Autodesk Inventor part; units mm, degrees
note: some values were not read from the file. Chosen so that the rebuilt part matches the saved one: direction of "Hole2".
(part 10 of 20)
  spline S30 degree 3 poles (-104.40532, -7.588503) (-104.41874, -7.589584) (-104.445196, -7.591715) (-104.484317, -7.593794) (-104.522133, -7.594934) (-104.558443, -7.595019) (-104.593058, -7.594014) (-104.625838, -7.591886) (-104.656702, -7.588699) (-104.685607, -7.584504) (-104.712509, -7.579351) (-104.737369, -7.573293) (-104.760145, -7.566381) (-104.780816, -7.55866) (-104.799541, -7.55008) (-104.816468, -7.540524) (-104.831907, -7.530078) (-104.841054, -7.522069) (-104.845542, -7.518139) knots 0 0 0 0 0.08847523 0.17442408 0.25743028 0.33708941 0.41301484 0.48496567 0.5529194 0.61687848 0.67685349 0.73286663 0.78495643 0.83318442 0.87777974 0.92016243 0.96082909 1 1 1 1
  ellipse E254 centre (-100.14545, -8.274184) end of major axis (-105.576804, -7.705925) minor radius 0.000387 (-103.277546, -7.946168) -> (-105.576804, -7.705925) ccw
  line L389 (-105.263014, -7.451577) -> (-105.576804, -7.705925)
  line L390 (-105.635035, -8.262493) -> (-105.576804, -7.705925)
  spline S31 degree 3 poles (-100.151462, -7.809621) (-100.108876, -7.785381) (-100.024585, -7.737401) (-99.898341, -7.668093) (-99.77384, -7.601642) (-99.611401, -7.517822) (-99.411986, -7.419431) (-99.251066, -7.347613) (-99.172025, -7.312337) knots 0 0 0 0 0.13376268 0.26475964 0.39312605 0.51899363 0.76373828 1 1 1 1
  line L391 (-100.151462, -7.991347) -> (-100.151462, -7.809621)
  line L392 (-93.85162, -7.809621) -> (-93.85162, -7.991347)
  spline S32 degree 3 poles (-94.831057, -7.312337) (-94.752016, -7.347613) (-94.591096, -7.419431) (-94.391681, -7.517822) (-94.229242, -7.601642) (-94.104741, -7.668093) (-93.978497, -7.737401) (-93.894206, -7.785381) (-93.85162, -7.809621) knots 0 0 0 0 0.23626172 0.48100637 0.60687395 0.73524036 0.86623732 1 1 1 1
  line L393 (-99.172025, -7.312337) -> (-94.831057, -7.312337)
  ellipse E255 centre (-97.001541, -7.776601) end of major axis (-101.962541, -7.776601) minor radius 0.5163 (-94.326958, -7.341758) -> (-94.831057, -7.312337) ccw
  ellipse E256 centre (-97.001541, -7.776601) end of major axis (-101.962541, -7.776601) minor radius 0.5163 (-99.172025, -7.312337) -> (-99.676124, -7.341758) ccw
  ellipse E257 centre (-97.001541, -8.273886) end of major axis (-91.540541, -8.273886) minor radius 0.568336 (-91.704205, -8.135789) -> (-93.85162, -7.809621) ccw
  ellipse E258 centre (-97.001541, -8.273886) end of major axis (-102.462541, -8.273886) minor radius 0.568336 (-100.151462, -7.809621) -> (-102.298877, -8.135789) ccw
  line L394 (-90.725538, -7.946169) -> (-90.670456, -8.472633)
  spline S33 degree 3 poles (-91.751687, -7.550801) (-91.669382, -7.577853) (-91.501806, -7.632932) (-91.293188, -7.71057) (-91.122866, -7.777485) (-90.992088, -7.830981) (-90.859278, -7.887152) (-90.770428, -7.926359) (-90.725538, -7.946169) knots 0 0 0 0 0.23621694 0.48094583 0.60681683 0.73519436 0.86621031 1 1 1 1
  spline S34 degree 3 poles (-89.157988, -7.517944) (-89.162657, -7.521949) (-89.172225, -7.530157) (-89.188451, -7.540872) (-89.206369, -7.550757) (-89.226095, -7.559652) (-89.247576, -7.567587) (-89.270807, -7.574535) (-89.295769, -7.580486) (-89.322449, -7.585424) (-89.350849, -7.589337) (-89.381017, -7.592209) (-89.412986, -7.594055) (-89.446759, -7.594893) (-89.48228, -7.594733) (-89.519486, -7.593567) (-89.558321, -7.59147) (-89.584711, -7.589321) (-89.598176, -7.588225) knots 0 0 0 0 0.04039145 0.08278851 0.12750015 0.17478558 0.22486002 0.27790108 0.33405492 0.39344169 0.45616024 0.52241148 0.59256068 0.66658365 0.74441779 0.82598879 0.91121312 1 1 1 1
  ellipse E259 centre (-93.857632, -8.274184) end of major axis (-88.426278, -7.705925) minor radius 0.000387 (-88.426278, -7.705925) -> (-90.725538, -7.946169) ccw
  line L395 (-88.740068, -7.451577) -> (-88.426278, -7.705925)
  line L396 (-88.368047, -8.262493) -> (-88.426278, -7.705925)
  spline S35 degree 3 poles (-102.805515, -6.019471) (-102.76082, -5.999226) (-102.672356, -5.959154) (-102.540099, -5.901692) (-102.409849, -5.846925) (-102.240187, -5.778353) (-102.032335, -5.698687) (-101.865304, -5.641978) (-101.783267, -5.614125) knots 0 0 0 0 0.13378969 0.26480564 0.39318317 0.51905417 0.76378306 1 1 1 1
  line L397 (-102.975863, -7.816663) -> (-102.805515, -6.019471)
  line L398 (-101.783267, -5.614125) -> (-100.987533, -5.689549)
  ellipse E260 centre (-99.622787, -5.818958) end of major axis (-104.561651, -5.350823) minor radius 0.000055 (-104.391855, -5.366902) -> (-104.561651, -5.350823) ccw
  ellipse E261 centre (-99.622787, -5.818958) end of major axis (-104.561651, -5.350823) minor radius 0.000055 (-101.783266, -5.614125) -> (-103.1187, -5.487555) ccw
  spline S36 degree 3 poles (-103.1187, -5.487555) (-103.170269, -5.503399) (-103.271281, -5.534435) (-103.420651, -5.575305) (-103.563643, -5.610313) (-103.699415, -5.638784) (-103.82825, -5.660668) (-103.949867, -5.675145) (-104.046402, -5.680859) (-104.118031, -5.680505) (-104.166268, -5.677754) (-104.210339, -5.672689) (-104.25009, -5.665479) (-104.285402, -5.656276) (-104.324871, -5.642155) (-104.366212, -5.619321) (-104.403393, -5.581425) (-104.424361, -5.534093) (-104.426921, -5.48054) (-104.415741, -5.423604) (-104.400067, -5.386398) (-104.391854, -5.366903) knots 0 0 0 0 0.10413454 0.20397599 0.29888876 0.38827472 0.47171081 0.55106733 0.62459732 0.65820388 0.68929134 0.71781594 0.74378428 0.76721832 0.78816557 0.82463321 0.85738378 0.88888098 0.92222056 0.95924484 1 1 1 1
  ellipse E262 centre (-99.669969, -6.316727) end of major axis (-105.106601, -5.80141) minor radius 0.000061 (-102.805556, -6.019467) -> (-105.106601, -5.80141) ccw
  line L399 (-104.561651, -5.350823) -> (-105.106601, -5.80141)
  ellipse E263 centre (-103.06077, -5.493063) end of major axis (-101.556214, -5.635674) minor radius 0.000017 (-104.392312, -5.366859) -> (-103.201425, -5.479748) ccw
  line L400 (-105.263014, -7.451577) -> (-105.106601, -5.80141)
  spline S37 degree 3 poles (-100.151462, -5.895967) (-100.108876, -5.871702) (-100.024586, -5.823676) (-99.898342, -5.7543) (-99.77384, -5.687785) (-99.611402, -5.603883) (-99.411989, -5.505397) (-99.251066, -5.433507) (-99.172025, -5.398196) knots 0 0 0 0 0.13376751 0.26476787 0.39313627 0.51900446 0.76374629 1 1 1 1
  line L401 (-100.151462, -7.610065) -> (-100.151462, -5.895967)
  line L402 (-93.85162, -5.895967) -> (-93.85162, -7.610065)
  spline S38 degree 3 poles (-94.831057, -5.398196) (-94.752016, -5.433507) (-94.591094, -5.505397) (-94.39168, -5.603883) (-94.229242, -5.687785) (-94.10474, -5.7543) (-93.978496, -5.823676) (-93.894206, -5.871702) (-93.85162, -5.895967) knots 0 0 0 0 0.23625371 0.48099554 0.60686373 0.73523213 0.86623249 1 1 1 1
  line L403 (-99.172025, -5.398196) -> (-94.831057, -5.398196)
  ellipse E264 centre (-97.001541, -5.81898) end of major axis (-101.962541, -5.81898) minor radius 0.467946 (-93.489707, -5.488458) -> (-94.831057, -5.398196) ccw
  ellipse E265 centre (-97.001541, -5.81898) end of major axis (-101.962541, -5.81898) minor radius 0.467946 (-99.172025, -5.398196) -> (-100.513375, -5.488458) ccw
  spline S39 degree 3 poles (-100.513375, -5.488458) (-100.553469, -5.506646) (-100.632452, -5.542475) (-100.749826, -5.59336) (-100.863732, -5.640862) (-100.973727, -5.684603) (-101.079308, -5.724356) (-101.180707, -5.760154) (-101.278249, -5.791822) (-101.371464, -5.819065) (-101.458467, -5.841159) (-101.537132, -5.857069) (-101.605936, -5.86658) (-101.66404, -5.870073) (-101.71224, -5.867867) (-101.750939, -5.859466) (-101.782429, -5.845833) (-101.795976, -5.830244) (-101.802272, -5.822999) knots 0 0 0 0 0.09648314 0.19006443 0.28034292 0.36693478 0.44946267 0.527566 0.60257164 0.67417927 0.74035842 0.79922956 0.84998037 0.89243012 0.92670891 0.95522625 0.97919149 1 1 1 1
  spline S40 degree 3 poles (-92.200822, -5.822993) (-92.206969, -5.830063) (-92.220263, -5.845354) (-92.251449, -5.858818) (-92.290121, -5.867201) (-92.337694, -5.869807) (-92.393667, -5.866938) (-92.458256, -5.858357) (-92.531448, -5.843945) (-92.613159, -5.823884) (-92.702907, -5.798329) (-92.799966, -5.7675) (-92.903601, -5.73162) (-93.013071, -5.690938) (-93.127471, -5.645689) (-93.287624, -5.579321) (-93.408219, -5.525098) (-93.489707, -5.488458) knots 0 0 0 0 0.02031374 0.04393674 0.07255557 0.10706143 0.14790384 0.19530387 0.24973648 0.31134419 0.37967367 0.4542385 0.53453299 0.62003981 0.71019877 0.8041769 1 1 1 1
  ellipse E266 centre (-97.001541, -6.31675) end of major axis (-91.540541, -6.31675) minor radius 0.515109 (-91.846496, -6.146755) -> (-93.85162, -5.895967) ccw
  ellipse E267 centre (-97.001541, -6.31675) end of major axis (-102.462541, -6.31675) minor radius 0.515109 (-100.151462, -5.895967) -> (-102.156586, -6.146755) ccw
  line L404 (-91.197567, -6.019471) -> (-91.027219, -7.816663)
  spline S41 degree 3 poles (-92.219815, -5.614125) (-92.137778, -5.641978) (-91.970747, -5.698687) (-91.762895, -5.778353) (-91.593233, -5.846925) (-91.462983, -5.901692) (-91.330726, -5.959154) (-91.242262, -5.999226) (-91.197567, -6.019471) knots 0 0 0 0 0.23621694 0.48094583 0.60681683 0.73519436 0.86621031 1 1 1 1
  line L405 (-93.015549, -5.689549) -> (-92.219815, -5.614125)
  ellipse E268 centre (-94.380295, -5.818958) end of major axis (-99.319158, -6.287094) minor radius 0.000055 (-90.882926, -5.487417) -> (-92.217961, -5.613949) ccw
  ellipse E269 centre (-94.380295, -5.818958) end of major axis (-89.441431, -5.350823) minor radius 0.000055 (-89.441431, -5.350823) -> (-89.611229, -5.366903) ccw
  spline S42 degree 3 poles (-89.611228, -5.366903) (-89.60278, -5.386911) (-89.58692, -5.424476) (-89.576014, -5.481491) (-89.57887, -5.534018) (-89.599249, -5.58047) (-89.636222, -5.618081) (-89.687727, -5.646719) (-89.753078, -5.66689) (-89.832365, -5.678643) (-89.925655, -5.681717) (-90.032585, -5.676653) (-90.152204, -5.663557) (-90.283105, -5.6426) (-90.423788, -5.613964) (-90.572421, -5.577931) (-90.727128, -5.535824) (-90.83142, -5.503812) (-90.884382, -5.487555) knots 0 0 0 0 0.04184874 0.07857029 0.11114659 0.14190435 0.17426777 0.21118388 0.25459927 0.30565856 0.36551927 0.43456112 0.51220716 0.59775966 0.69045627 0.7893544 0.8930296 1 1 1 1
  ellipse E270 centre (-94.333113, -6.316727) end of major axis (-88.896481, -5.80141) minor radius 0.000061 (-88.896481, -5.80141) -> (-91.197567, -6.019471) ccw
  line L406 (-89.441431, -5.350823) -> (-88.896481, -5.80141)
  line L407 (-88.740068, -7.451577) -> (-88.896481, -5.80141)
  ellipse E271 centre (-99.833277, -5.290471) end of major axis (-103.727023, -4.883084) minor radius 0.000278 (-100.192976, -5.252559) -> (-101.457275, -5.120305) ccw
  ellipse E272 centre (-101.772205, -5.087396) end of major axis (-101.57329, -5.108208) minor radius 0.000014 (-101.663429, -5.098789) -> (-101.57329, -5.108208) ccw
  line L408 (-101.573227, -5.108186) -> (-101.57329, -5.108208)
  ellipse E273 centre (-101.374312, -5.128998) end of major axis (-101.573227, -5.108186) minor radius 0.000014 (-101.457275, -5.120305) -> (-101.573227, -5.108186) ccw
  ellipse E274 centre (-99.833277, -5.290471) end of major axis (-103.180009, -4.940316) minor radius 0.000239 (-101.663429, -5.098789) -> (-103.180009, -4.940316) ccw
  line L409 (-103.180009, -4.940316) -> (-103.236104, -5.476461)
  ellipse E275 centre (-98.189163, 10.423755) end of major axis (-100.436894, 10.658926) minor radius 0.00016 (-100.162743, 10.63032) -> (-100.436894, 10.658926) ccw
  line L410 (-100.436894, 10.658926) -> (-100.733258, 8.711817)
  line L411 (-95.251541, -5.398196) -> (-95.251541, -4.938809)
  ellipse E276 centre (-95.451541, -4.938809) end of major axis (-95.251541, -4.938809) minor radius 0.020814 (-95.251541, -4.938809) -> (-95.368096, -4.919893) ccw
  ellipse E277 centre (-97.001541, -5.290177) end of major axis (-100.916541, -5.290177) minor radius 0.407441 (-95.368096, -4.919893) -> (-98.634987, -4.919893) ccw
  ellipse E278 centre (-95.051541, -4.979583) end of major axis (-95.251541, -4.979583) minor radius 0.020814 (-95.251541, -4.979583) -> (-95.160938, -4.997008) ccw
  ellipse E279 centre (-98.951541, -4.979583) end of major axis (-98.751541, -4.979583) minor radius 0.020814 (-98.842144, -4.997008) -> (-98.751541, -4.979583) ccw
  ellipse E280 centre (-98.551541, -4.938809) end of major axis (-98.751541, -4.938809) minor radius 0.020814 (-98.634987, -4.919893) -> (-98.751541, -4.938809) ccw
  line L412 (-98.751541, -4.938809) -> (-98.751541, -5.398196)
  ellipse E281 centre (-97.001541, -5.290177) end of major axis (-93.636541, -5.290177) minor radius 0.350202 (-93.673685, -5.238287) -> (-95.160938, -4.997008) ccw
  ellipse E282 centre (-97.001541, -5.290177) end of major axis (-100.366541, -5.290177) minor radius 0.350202 (-98.842144, -4.997008) -> (-100.329397, -5.238287) ccw
  ellipse E283 centre (-97.001541, 10.424026) end of major axis (-94.741541, 10.424026) minor radius 0.235202 (-95.963463, 10.632949) -> (-98.039619, 10.632949) ccw
  ellipse E284 centre (-92.62877, -5.128998) end of major axis (-92.429855, -5.108186) minor radius 0.000014 (-92.429855, -5.108186) -> (-92.545807, -5.120305) ccw
  ellipse E285 centre (-94.169805, -5.290471) end of major axis (-98.063552, -5.697857) minor radius 0.000278 (-92.545794, -5.120304) -> (-93.810092, -5.252558) ccw
  line L413 (-92.429792, -5.108208) -> (-92.429855, -5.108186)
  ellipse E286 centre (-92.230877, -5.087396) end of major axis (-92.429792, -5.108208) minor radius 0.000014 (-92.429792, -5.108208) -> (-92.339653, -5.098789) ccw
  ellipse E287 centre (-94.169805, -5.290471) end of major axis (-90.823073, -4.940316) minor radius 0.000239 (-90.823073, -4.940316) -> (-92.339656, -5.098789) ccw
  line L414 (-90.823073, -4.940316) -> (-90.766978, -5.476461)
  ellipse E288 centre (-95.813919, 10.423755) end of major axis (-93.566188, 10.658926) minor radius 0.00016 (-93.566188, 10.658926) -> (-93.840339, 10.63032) ccw
  line L415 (-93.566188, 10.658926) -> (-93.269824, 8.711817)
  ellipse E289 centre (-98.540762, 8.455629) end of major axis (-100.785493, 8.717896) minor radius 0.000114 (-100.027352, 8.629403) -> (-100.785493, 8.717896) ccw
  line L416 (-100.785493, 8.717896) -> (-102.716328, -3.014524)
  line L417 (-102.765192, -3.311436) -> (-103.035733, -4.955341)
  ellipse E290 centre (-97.001541, -7.237173) end of major axis (-100.916541, -7.237173) minor radius 0.45382 (-96.283175, -6.791059) -> (-96.387015, -6.788979) ccw
  ellipse E291 centre (-97.001541, -7.237173) end of major axis (-100.916541, -7.237173) minor radius 0.45382 (-96.660869, -6.785075) -> (-97.397172, -6.785677) ccw
  ellipse E292 centre (-97.001541, -7.237173) end of major axis (-100.916541, -7.237173) minor radius 0.45382 (-97.616067, -6.788979) -> (-97.719907, -6.791059) ccw
  ellipse E293 centre (-97.001541, 8.456315) end of major axis (-94.741541, 8.456315) minor radius 0.261975 (-95.29258, 8.627743) -> (-98.710502, 8.627743) ccw
  ellipse E294 centre (-95.46232, 8.455629) end of major axis (-93.217589, 8.717896) minor radius 0.000114 (-93.217589, 8.717896) -> (-93.97573, 8.629403) ccw
  line L418 (-93.217589, 8.717896) -> (-91.286754, -3.014524)
  line L419 (-91.237891, -3.311436) -> (-90.967349, -4.955341)
  ellipse E295 centre (-97.802609, 13.384052) end of major axis (-97.598523, 13.364708) minor radius 0.000002 (-97.598523, 13.364708) -> (-97.844396, 13.388016) ccw
  ellipse E296 centre (-97.843747, 12.950044) end of major axis (-99.073236, 13.066582) minor radius 0.000014 (-98.187182, 12.98261) -> (-99.073236, 13.066582) ccw
  line L420 (-99.073236, 13.066582) -> (-99.125429, 12.515944)
  arc A2 (-98.1701, 13.394511) -> (-99.073236, 13.066582) centre (-97.983698, 11.473542) ccw
  arc A3 (-97.492698, 13.340033) -> (-97.598523, 13.364708) centre (-97.983698, 11.473542) ccw
  ellipse E297 centre (-99.386879, -3.330114) end of major axis (-103.28441, -2.960682) minor radius 0.000044 (-100.024938, -3.269591) -> (-101.012782, -3.175961) ccw
  ellipse E298 centre (-99.481243, -4.325652) end of major axis (-103.378773, -3.95622) minor radius 0.000044 (-99.731659, -4.301872) -> (-101.107145, -4.171499) ccw
  line L421 (-101.128829, -3.164963) -> (-101.128857, -3.164965)
  line L422 (-101.223192, -4.160501) -> (-101.22322, -4.160503)
  ellipse E299 centre (-99.386879, -3.330114) end of major axis (-102.736864, -3.012582) minor radius 0.000037 (-101.219068, -3.156416) -> (-102.736864, -3.012582) ccw
  ellipse E300 centre (-99.481243, -4.325652) end of major axis (-102.831227, -4.00812) minor radius 0.000037 (-101.31343, -4.151954) -> (-102.589961, -4.030974) ccw
  line L423 (-102.736864, -3.012582) -> (-102.765192, -3.31144)
  ellipse E301 centre (-97.895941, 12.399384) end of major axis (-100.145857, 12.612645) minor radius 0.000025 (-98.980833, 12.502239) -> (-100.145857, 12.612645) ccw
  line L424 (-100.145857, 12.612645) -> (-100.423969, 10.657591)
  ellipse E302 centre (-97.001541, 12.950091) end of major axis (-95.766541, 12.950091) minor radius 0.116491 (-95.815873, 12.982686) -> (-98.187209, 12.982686) ccw
  arc A4 (-97.205699, 13.392747) -> (-97.983204, 13.135272) centre (-97.001541, 11.473583) ccw
  arc A5 (-96.019879, 13.135272) -> (-96.797384, 13.392747) centre (-97.001541, 11.473583) ccw
  ellipse E303 centre (-95.451541, -4.007208) end of major axis (-95.251541, -4.007208) minor radius 0.018865 (-95.251541, -4.007208) -> (-95.368096, -3.990063) ccw
  line L425 (-95.251541, -4.007208) -> (-95.251541, -3.011666)
  ellipse E304 centre (-95.451541, -3.011666) end of major axis (-95.251541, -3.011666) minor radius 0.018865 (-95.251541, -3.011666) -> (-95.368096, -2.994522) ccw
  ellipse E305 centre (-97.001541, -3.330126) end of major axis (-100.916541, -3.330126) minor radius 0.369282 (-95.368096, -2.994522) -> (-98.634987, -2.994522) ccw
  ellipse E306 centre (-97.001541, -4.325668) end of major axis (-100.916541, -4.325668) minor radius 0.369282 (-95.368096, -3.990063) -> (-98.634987, -3.990063) ccw
  ellipse E307 centre (-95.051541, -3.048621) end of major axis (-95.251541, -3.048621) minor radius 0.018865 (-95.251541, -3.048621) -> (-95.160938, -3.064414) ccw
  ellipse E308 centre (-98.951541, -3.048621) end of major axis (-98.751541, -3.048621) minor radius 0.018865 (-98.842144, -3.064414) -> (-98.751541, -3.048621) ccw
  ellipse E309 centre (-98.551541, -3.011666) end of major axis (-98.751541, -3.011666) minor radius 0.018865 (-98.634987, -2.994522) -> (-98.751541, -3.011666) ccw
  ellipse E310 centre (-98.551541, -4.007208) end of major axis (-98.751541, -4.007208) minor radius 0.018865 (-98.634987, -3.990063) -> (-98.751541, -4.007208) ccw
  line L426 (-98.751541, -3.011666) -> (-98.751541, -4.007208)
  ellipse E311 centre (-95.051541, -4.044163) end of major axis (-95.251541, -4.044163) minor radius 0.018865 (-95.251541, -4.044163) -> (-95.160938, -4.059955) ccw
  line L427 (-95.251541, -4.044163) -> (-95.251541, -4.007208)
  ellipse E312 centre (-98.951541, -4.044163) end of major axis (-98.751541, -4.044163) minor radius 0.018865 (-98.842144, -4.059955) -> (-98.751541, -4.044163) ccw
  line L428 (-98.751541, -4.007208) -> (-98.751541, -4.044163)
  ellipse E313 centre (-97.001541, -3.330126) end of major axis (-93.636541, -3.330126) minor radius 0.317404 (-93.750966, -3.248059) -> (-95.160938, -3.064414) ccw
  ellipse E314 centre (-97.001541, -3.330126) end of major axis (-100.366541, -3.330126) minor radius 0.317404 (-98.842144, -3.064414) -> (-100.252116, -3.248059) ccw
  ellipse E315 centre (-97.001541, -4.325668) end of major axis (-100.366541, -4.325668) minor radius 0.317404 (-100.271387, -4.25072) -> (-100.340805, -4.286487) ccw
  ellipse E316 centre (-97.001541, -4.325668) end of major axis (-93.636541, -4.325668) minor radius 0.317404 (-98.842144, -4.059955) -> (-100.062388, -4.1938) ccw
  ellipse E317 centre (-97.001541, -4.325668) end of major axis (-93.636541, -4.325668) minor radius 0.317404 (-93.940694, -4.1938) -> (-95.160938, -4.059955) ccw
  ellipse E318 centre (-97.001541, -4.325668) end of major axis (-93.636541, -4.325668) minor radius 0.317404 (-93.662277, -4.286487) -> (-93.731695, -4.25072) ccw
  ellipse E319 centre (-97.001541, 12.399429) end of major axis (-94.741541, 12.399429) minor radius 0.213175 (-95.021924, 12.50227) -> (-98.981158, 12.50227) ccw
  ellipse E320 centre (-96.200474, 13.384052) end of major axis (-96.404559, 13.364708) minor radius 0.000002 (-96.158686, 13.388016) -> (-96.404559, 13.364708) ccw
  ellipse E321 centre (-96.159336, 12.950044) end of major axis (-94.929846, 13.066582) minor radius 0.000014 (-94.929846, 13.066582) -> (-95.8159, 12.98261) ccw
  line L429 (-94.929846, 13.066582) -> (-94.877653, 12.515944)
  arc A6 (-96.404559, 13.364708) -> (-96.510384, 13.340033) centre (-96.019384, 11.473542) ccw
  arc A7 (-94.929846, 13.066582) -> (-95.832982, 13.394511) centre (-96.019384, 11.473542) ccw
  ellipse E322 centre (-94.616203, -3.330114) end of major axis (-98.513733, -3.699546) minor radius 0.000044 (-92.989786, -3.175912) -> (-93.977586, -3.269538) ccw
  ellipse E323 centre (-94.521839, -4.325652) end of major axis (-98.41937, -4.695083) minor radius 0.000044 (-92.895423, -4.17145) -> (-94.270859, -4.301818) ccw
  line L430 (-92.874225, -3.164965) -> (-92.874253, -3.164963)
  line L431 (-92.779862, -4.160503) -> (-92.77989, -4.160501)
  ellipse E324 centre (-94.616203, -3.330114) end of major axis (-91.266218, -3.012582) minor radius 0.000037 (-91.266218, -3.012582) -> (-92.784108, -3.156425) ccw
  ellipse E325 centre (-94.521839, -4.325652) end of major axis (-91.171855, -4.00812) minor radius 0.000037 (-91.41312, -4.030974) -> (-92.68965, -4.151954) ccw
  line L432 (-91.266218, -3.012582) -> (-91.23789, -3.31144)
  ellipse E326 centre (-96.107141, 12.399384) end of major axis (-93.857225, 12.612645) minor radius 0.000025 (-93.857225, 12.612645) -> (-95.022249, 12.502239) ccw
  line L433 (-93.857225, 12.612645) -> (-93.579113, 10.657591)
  line L434 (-89.836306, -39.801561) -> (-90.501958, -38.086358)
  line L435 (-87.761586, -39.801561) -> (-88.303845, -37.920957)
  line L436 (-106.795587, -39.801561) -> (-106.897672, -37.782333)
  line L437 (-104.725301, -39.801561) -> (-104.622766, -37.850618)
  line L438 (-89.880813, -39.139047) -> (-90.11399, -38.038909)
  line L439 (-87.749763, -39.085429) -> (-87.891287, -37.830541)
  line L440 (-106.253319, -39.085429) -> (-106.111795, -37.830541)
  line L441 (-104.12227, -39.139047) -> (-103.889092, -38.038909)
  line L442 (-89.277781, -39.801561) -> (-89.380316, -37.850618)
  line L443 (-87.207496, -39.801561) -> (-87.106374, -37.801401)
  line L444 (-106.241496, -39.801561) -> (-105.696994, -37.913178)
  line L445 (-104.166776, -39.801561) -> (-103.501124, -38.086358)
  line L446 (-89.601791, -38.390849) -> (-89.684484, -37.945244)
  line L447 (-87.415885, -38.40542) -> (-87.476578, -37.784138)
  line L448 (-106.587197, -38.40542) -> (-106.526504, -37.784138)
  line L449 (-104.401292, -38.390849) -> (-104.318598, -37.945244)
  ellipse E327 centre (-107.424482, -24.551038) end of major axis (-107.497848, -24.375774) minor radius 0.172083 (-107.599289, -24.542874) -> (-107.493364, -24.717688) ccw
  ellipse E328 centre (-107.483138, -24.575592) end of major axis (-107.409772, -24.750856) minor radius 0.172083 (-107.618457, -24.683795) -> (-107.56024, -24.737582) ccw
  ellipse E329 centre (-107.413108, -27.354914) end of major axis (-107.486474, -27.17965) minor radius 0.172083 (-107.525342, -27.203052) -> (-107.545513, -27.222774) ccw
  ellipse E330 centre (-107.674507, -24.573932) end of major axis (-107.683372, -24.763725) minor radius 0.073999 (-107.669789, -24.761191) -> (-107.600209, -24.542831) ccw
  ellipse E331 centre (-107.812513, -24.567486) end of major axis (-107.821377, -24.757279) minor radius 0.073999 (-107.807794, -24.754746) -> (-107.738215, -24.536385) ccw
  ellipse E332 centre (-107.742483, -27.346808) end of major axis (-107.733618, -27.157015) minor radius 0.073999 (-107.668184, -27.315707) -> (-107.747201, -27.159549) ccw
  ellipse E333 centre (-107.354452, -27.33036) end of major axis (-107.427818, -27.155096) minor radius 0.172083 (-107.458618, -27.172309) -> (-107.529259, -27.322196) ccw
  ellipse E334 centre (-107.604477, -27.353254) end of major axis (-107.595612, -27.163461) minor radius 0.073999 (-107.530179, -27.322153) -> (-107.595612, -27.163461) ccw
  line L450 (-107.595612, -27.163461) -> (-107.733618, -27.157015)
  line L451 (-107.320508, -24.770227) -> (-107.411556, -24.765974)
  line L452 (-107.337736, -24.742129) -> (-107.218796, -24.747684)
  line L453 (-106.733437, -27.012581) -> (-106.744387, -26.578006)
  line L454 (-106.779637, -25.17899) -> (-106.784594, -24.982296)
  line L455 (-108.045478, -24.854241) -> (-107.807794, -24.754746)
  line L456 (-107.669789, -24.761191) -> (-107.800448, -24.815885)
  line L457 (-107.747201, -27.159549) -> (-107.847783, -27.201653)
  line L458 (-108.068664, -27.10488) -> (-108.119821, -25.074595)
  line L459 (-107.151556, -27.152798) -> (-107.232991, -27.148994)
  line L460 (-107.981815, -25.081041) -> (-107.930658, -27.111326)
  line L461 (-106.725937, -24.957742) -> (-106.720023, -25.192452)
  line L462 (-106.694116, -26.22064) -> (-106.67478, -26.988027)
  ellipse E335 centre (-107.517905, -23.195787) end of major axis (-107.591271, -23.020523) minor radius 0.172083 (-107.591271, -23.020523) -> (-107.650311, -23.063647) ccw
  ellipse E336 centre (-107.378341, -28.734719) end of major axis (-107.304975, -28.909983) minor radius 0.172083 (-107.51366, -28.842922) -> (-107.50192, -28.857667) ccw
  ellipse E337 centre (-107.319685, -28.710166) end of major axis (-107.393051, -28.534902) minor radius 0.172083 (-107.494492, -28.702001) -> (-107.434983, -28.842027) ccw
  ellipse E338 centre (-107.459249, -23.171233) end of major axis (-107.532615, -22.995969) minor radius 0.172083 (-107.51781, -22.990633) -> (-107.634056, -23.163068) ccw
  line L463 (-107.591271, -23.020523) -> (-107.532615, -22.995969)
  line L464 (-107.351927, -28.922992) -> (-106.338665, -28.970317)
  line L465 (-107.494492, -28.702001) -> (-107.529259, -27.322196)
  line L466 (-106.927292, -28.915532) -> (-107.278106, -28.899146)
  line L467 (-107.250149, -22.99396) -> (-107.201576, -22.996229)
  line L468 (-107.599289, -24.542874) -> (-107.634056, -23.163068)
  ellipse E339 centre (-106.908244, -27.004416) end of major axis (-106.834878, -27.17968) minor radius 0.172083 (-106.768249, -27.127038) -> (-106.733437, -27.012581) ccw
  ellipse E340 centre (-106.959401, -24.974131) end of major axis (-106.886035, -25.149395) minor radius 0.172083 (-106.784594, -24.982296) -> (-106.792606, -24.930572) ccw
  ellipse E341 centre (-107.994366, -27.073779) end of major axis (-108.00323, -27.263572) minor radius 0.073999 (-108.068664, -27.10488) -> (-108.052515, -27.206678) ccw
  ellipse E342 centre (-108.045523, -25.043494) end of major axis (-108.036658, -24.853701) minor radius 0.073999 (-108.063135, -24.864536) -> (-108.119821, -25.074595) ccw
  ellipse E343 centre (-106.900744, -24.949578) end of major axis (-106.97411, -24.774314) minor radius 0.172083 (-106.725937, -24.957742) -> (-106.753988, -24.858996) ccw
  ellipse E344 centre (-106.849587, -26.979863) end of major axis (-106.776221, -27.155126) minor radius 0.172083 (-106.734412, -27.129255) -> (-106.67478, -26.988027) ccw
  ellipse E345 centre (-107.85636, -27.080224) end of major axis (-107.847495, -26.890431) minor radius 0.073999 (-107.930658, -27.111326) -> (-107.920556, -27.192393) ccw
  ellipse E346 centre (-107.907517, -25.049939) end of major axis (-107.898652, -24.860146) minor radius 0.073999 (-107.97813, -25.008291) -> (-107.981815, -25.081041) ccw
  line L469 (-107.738215, -24.536385) -> (-107.772982, -23.15658)
  line L470 (-107.851998, -23.000422) -> (-108.036921, -23.077831)
  line L471 (-108.14986, -29.100931) -> (-107.702997, -28.913873)
  line L472 (-107.633418, -28.695512) -> (-107.668184, -27.315707)
  line L473 (-107.600209, -24.542831) -> (-107.634976, -23.163025)
  line L474 (-107.495412, -28.701958) -> (-107.530179, -27.322153)
  line L475 (-108.417464, -29.277166) -> (-107.564992, -28.920319)
  ellipse E347 centre (-107.84728, -23.187681) end of major axis (-107.838415, -22.997888) minor radius 0.073999 (-107.772982, -23.15658) -> (-107.851998, -23.000422) ccw
  ellipse E348 centre (-107.707716, -28.726614) end of major axis (-107.71658, -28.916407) minor radius 0.073999 (-107.702997, -28.913873) -> (-107.633418, -28.695512) ccw
  ellipse E349 centre (-107.709274, -23.194127) end of major axis (-107.70041, -23.004334) minor radius 0.073999 (-107.634976, -23.163025) -> (-107.70041, -23.004334) ccw
  ellipse E350 centre (-107.56971, -28.733059) end of major axis (-107.578575, -28.922853) minor radius 0.073999 (-107.564992, -28.920319) -> (-107.495412, -28.701958) ccw
  line L476 (-107.838415, -22.997888) -> (-107.70041, -23.004334)
  line L477 (-107.648967, -29.358549) -> (-108.285216, -29.328832)
  line L478 (-108.343872, -29.353386) -> (-107.647584, -29.385907)
  ellipse E351 centre (-108.187455, -29.287909) end of major axis (-108.437376, -29.294207) minor radius 0.041852 (-108.417464, -29.277166) -> (-108.285216, -29.328832) ccw
  ellipse E352 centre (-108.187455, -29.287909) end of major axis (-108.587328, -29.297985) minor radius 0.066962 (-108.585467, -29.291196) -> (-108.343872, -29.353386) ccw
  line L479 (-108.587477, -29.292074) -> (-108.587328, -29.297985)
  line L480 (-87.560521, -24.714054) -> (-87.279601, -24.703624)
  line L481 (-87.428378, -26.95356) -> (-87.56132, -25.684022)
  ellipse E353 centre (-87.393205, -23.121791) end of major axis (-87.418109, -22.93343) minor radius 0.101721 (-87.313826, -23.0264) -> (-87.412975, -22.932997) ccw
  line L482 (-87.412975, -22.932997) -> (-87.516236, -22.93683)
  line L483 (-87.324785, -28.914822) -> (-87.030053, -28.903879)
  line L484 (-87.019614, -28.903492) -> (-86.951072, -28.900947)
  line L485 (-87.511613, -28.933701) -> (-87.405313, -28.929755)
  ellipse E354 centre (-87.326403, -26.949774) end of major axis (-87.301499, -27.138135) minor radius 0.101721 (-87.428378, -26.95356) -> (-87.338805, -27.130661) ccw
  ellipse E355 centre (-87.540751, -24.902848) end of major axis (-87.565655, -24.714488) minor radius 0.101721 (-87.560521, -24.714054) -> (-87.560874, -24.714068) ccw
  line L486 (-106.375782, -22.953277) -> (-106.465761, -22.953134)
  line L487 (-106.710484, -28.915657) -> (-106.670867, -28.91572)
  line L488 (-106.481887, -28.916019) -> (-106.25106, -28.916385)
  line L489 (-106.158165, -28.727707) -> (-106.085563, -28.034397)
  line L490 (-106.587235, -28.932506) -> (-106.518088, -28.932616)
  ellipse E356 centre (-106.23129, -28.727591) end of major axis (-106.254421, -28.916178) minor radius 0.072673 (-106.25106, -28.916385) -> (-106.158165, -28.727707) ccw
  line L491 (-106.219982, -27.147438) -> (-106.263661, -27.147368)
  ellipse E357 centre (-106.098926, -22.998128) end of major axis (-106.496751, -22.956469) minor radius 0.017093 (-106.465761, -22.953134) -> (-106.496751, -22.956469) ccw
  line L492 (-106.496751, -22.956469) -> (-106.497264, -22.961369)
  line L493 (-85.58781, -29.276018) -> (-85.977019, -29.308696)
  line L494 (-86.35471, -29.370329) -> (-85.506315, -29.299099)
  ellipse E358 centre (-85.583091, -29.088759) end of major axis (-85.634867, -29.271568) minor radius 0.156811 (-85.58781, -29.276018) -> (-85.503367, -29.241082) ccw
  ellipse E359 centre (-85.501597, -29.11184) end of major axis (-85.553373, -29.294649) minor radius 0.156811 (-85.506315, -29.299099) -> (-85.419544, -29.262283) ccw
  line L495 (-86.327432, -23.005815) -> (-86.358769, -22.996939)
  line L496 (-86.50777, -28.910391) -> (-86.068015, -29.03494)
  line L497 (-86.515336, -28.954467) -> (-85.449259, -29.256406)
  line L498 (-86.402973, -24.751263) -> (-86.087861, -24.840511)
  line L499 (-85.989353, -25.057006) -> (-86.04051, -27.087291)
  ellipse E360 centre (-86.738642, -24.779445) end of major axis (-86.338769, -24.789521) minor radius 0.066962 (-86.402973, -24.751263) -> (-86.627877, -24.717796) ccw
  line L500 (-87.36115, -24.751914) -> (-87.020704, -24.723331)
  ellipse E361 centre (-86.738642, -24.779445) end of major axis (-86.988563, -24.773148) minor radius 0.041852 (-86.754457, -24.737277) -> (-86.868524, -24.740497) ccw
  line L501 (-86.372358, -24.806153) -> (-86.437773, -24.787626)
  ellipse E362 centre (-86.799236, -27.184249) end of major axis (-87.199109, -27.174173) minor radius 0.066962 (-86.473415, -27.153396) -> (-86.748949, -27.119029) ccw
  line L502 (-87.458214, -24.97685) -> (-87.464599, -25.230258)
  ellipse E363 centre (-86.092579, -25.02777) end of major axis (-86.108475, -24.838436) minor radius 0.102463 (-85.989353, -25.057006) -> (-86.087861, -24.840511) ccw
  ellipse E364 centre (-86.143736, -27.058055) end of major axis (-86.159632, -26.868721) minor radius 0.102463 (-86.068434, -27.202124) -> (-86.04051, -27.087291) ccw
  ellipse E365 centre (-87.298771, -24.963464) end of major axis (-87.246995, -24.780654) minor radius 0.156811 (-87.447033, -24.912144) -> (-87.458214, -24.97685) ccw
  ellipse E366 centre (-87.380266, -24.940382) end of major axis (-87.432042, -25.123192) minor radius 0.156811 (-87.415314, -24.762322) -> (-87.5126, -24.851792) ccw
  line L503 (-87.666452, -28.957799) -> (-87.369579, -28.932874)
  line L504 (-87.037597, -28.905002) -> (-86.979263, -28.900104)
  ellipse E367 centre (-86.843439, -28.938573) end of major axis (-86.593519, -28.94487) minor radius 0.041852 (-86.834301, -28.89696) -> (-86.979263, -28.900104) ccw
  ellipse E368 centre (-86.694439, -23.025121) end of major axis (-87.094312, -23.015046) minor radius 0.066962 (-86.358769, -22.996939) -> (-86.662307, -22.959142) ccw
  ellipse E369 centre (-86.843439, -28.938573) end of major axis (-87.243312, -28.928497) minor radius 0.066962 (-86.50777, -28.910391) -> (-86.672405, -28.882215) ccw
  ellipse E370 centre (-85.444541, -29.069147) end of major axis (-85.428645, -29.258481) minor radius 0.102463 (-85.449259, -29.256406) -> (-85.430097, -29.258583) ccw
  line L505 (-87.934435, -29.313625) -> (-87.978745, -29.301075)
  ellipse E371 centre (-107.762483, -24.584082) end of major axis (-107.838534, -24.409967) minor radius 0.168992 (-107.934755, -24.578254) -> (-107.844467, -24.740213) ccw
  ellipse E372 centre (-107.825313, -24.611525) end of major axis (-107.749262, -24.785641) minor radius 0.168992 (-107.953508, -24.724161) -> (-107.902972, -24.770492) ccw
  ellipse E373 centre (-108.015245, -24.612984) end of major axis (-108.02167, -24.802875) minor radius 0.079929 (-108.005806, -24.799686) -> (-107.935661, -24.578223) ccw
  ellipse E374 centre (-108.151248, -24.608382) end of major axis (-108.157673, -24.798274) minor radius 0.079929 (-108.141809, -24.795085) -> (-108.071665, -24.573622) ccw
  ellipse E375 centre (-108.011153, -27.379437) end of major axis (-108.004728, -27.189545) minor radius 0.079929 (-107.931569, -27.344676) -> (-108.020592, -27.192735) ccw
  ellipse E376 centre (-107.622388, -27.355137) end of major axis (-107.698438, -27.181021) minor radius 0.168992 (-107.760634, -27.230947) -> (-107.794659, -27.349308) ccw
  ellipse E377 centre (-107.875149, -27.384038) end of major axis (-107.868725, -27.194147) minor radius 0.079929 (-107.795566, -27.349278) -> (-107.868725, -27.194147) ccw
  line L506 (-107.868725, -27.194147) -> (-108.004728, -27.189545)
  line L507 (-107.68574, -24.80263) -> (-107.762572, -24.800031)
  line L508 (-107.697218, -24.772673) -> (-107.621932, -24.775221)
  line L509 (-107.024984, -27.032151) -> (-107.043066, -26.674485)
  line L510 (-107.117621, -25.199823) -> (-107.127323, -25.007906)
  line L511 (-108.401503, -24.908514) -> (-108.141809, -24.795085)
  line L512 (-108.005806, -24.799686) -> (-108.2655, -24.913115)
  line L513 (-109.054927, -25.193917) -> (-108.811987, -25.087806)
  line L514 (-108.722964, -25.239747) -> (-108.620625, -27.263993)
  line L515 (-108.690769, -27.485456) -> (-108.933709, -27.591567)
  line L516 (-108.020592, -27.192735) -> (-108.280286, -27.306164)
  line L517 (-108.369308, -27.154222) -> (-108.471648, -25.129977)
  line L518 (-107.54667, -27.171316) -> (-107.577523, -27.170272)
  line L519 (-108.335644, -25.134578) -> (-108.233305, -27.158824)
  ellipse E378 centre (-108.69225, -25.206188) end of major axis (-109.09174, -25.226384) minor radius 0.071491 (-109.054927, -25.193917) -> (-108.859795, -25.279368) ccw
  line L520 (-108.720723, -25.284073) -> (-108.859795, -25.279368)
  line L521 (-108.796966, -25.251925) -> (-108.739316, -25.253876)
  ellipse E379 centre (-108.69225, -25.206188) end of major axis (-108.941932, -25.218811) minor radius 0.044682 (-108.918923, -25.198519) -> (-108.796966, -25.251925) ccw
  line L522 (-108.749355, -25.124455) -> (-108.918923, -25.198519)
  ellipse E380 centre (-108.571033, -27.603837) end of major axis (-108.970523, -27.624034) minor radius 0.071491 (-108.933709, -27.591567) -> (-108.970523, -27.624034) ccw
  line L523 (-107.064494, -24.980463) -> (-107.050174, -25.263715)
  line L524 (-106.979882, -26.654075) -> (-106.962155, -27.004709)
  ellipse E381 centre (-107.894864, -23.235824) end of major axis (-107.970914, -23.061708) minor radius 0.168992 (-107.970914, -23.061708) -> (-108.025062, -23.101615) ccw
  ellipse E382 centre (-107.615666, -28.75828) end of major axis (-107.539615, -28.932396) minor radius 0.168992 (-107.621064, -28.943791) -> (-107.606227, -28.944982) ccw
  ellipse E383 centre (-107.552837, -28.730837) end of major axis (-107.628887, -28.556722) minor radius 0.168992 (-107.557786, -28.916405) -> (-107.543398, -28.91754) ccw
  ellipse E384 centre (-107.552837, -28.730837) end of major axis (-107.628887, -28.556722) minor radius 0.168992 (-107.725108, -28.725009) -> (-107.707888, -28.798048) ccw
  ellipse E385 centre (-107.832035, -23.208382) end of major axis (-107.908085, -23.034266) minor radius 0.168992 (-107.90197, -23.031753) -> (-108.004306, -23.202553) ccw
  line L525 (-107.970914, -23.061708) -> (-107.908085, -23.034266)
  line L526 (-107.606227, -28.944982) -> (-107.589593, -28.945545)
  line L527 (-107.43766, -28.950685) -> (-106.344072, -28.987685)
  line L528 (-107.725108, -28.725009) -> (-107.794659, -27.349308)
  line L529 (-107.272232, -28.926714) -> (-107.354802, -28.923921)
  line L530 (-107.522928, -28.918232) -> (-107.543398, -28.91754)
  line L531 (-107.667141, -23.027578) -> (-107.649281, -23.028182)
  line L532 (-107.934755, -24.578254) -> (-108.004306, -23.202553)
  ellipse E386 centre (-107.197255, -27.026323) end of major axis (-107.121205, -27.200439) minor radius 0.168992 (-107.037955, -27.112598) -> (-107.024984, -27.032151) ccw
  ellipse E387 centre (-107.299595, -25.002077) end of major axis (-107.223544, -25.176193) minor radius 0.168992 (-107.127323, -25.007906) -> (-107.134695, -24.962669) ccw
  ellipse E388 centre (-108.802548, -25.274508) end of major axis (-108.796123, -25.084617) minor radius 0.079929 (-108.722964, -25.239747) -> (-108.811987, -25.087806) ccw
  ellipse E389 centre (-108.700209, -27.298753) end of major axis (-108.706633, -27.488645) minor radius 0.079929 (-108.690769, -27.485456) -> (-108.620625, -27.263993) ccw
  ellipse E390 centre (-108.289725, -27.119462) end of major axis (-108.296149, -27.309353) minor radius 0.079929 (-108.369308, -27.154222) -> (-108.280286, -27.306164) ccw
  ellipse E391 centre (-108.392064, -25.095216) end of major axis (-108.38564, -24.905325) minor radius 0.079929 (-108.401503, -24.908514) -> (-108.471648, -25.129977) ccw
  ellipse E392 centre (-107.236765, -24.974635) end of major axis (-107.312816, -24.800519) minor radius 0.168992 (-107.064494, -24.980463) -> (-107.070367, -24.940927) ccw
  ellipse E393 centre (-107.134426, -26.99888) end of major axis (-107.210476, -26.824764) minor radius 0.168992 (-106.996566, -27.123589) -> (-106.962155, -27.004709) ccw
  ellipse E394 centre (-108.153721, -27.124063) end of major axis (-108.147297, -26.934172) minor radius 0.079929 (-108.233305, -27.158824) -> (-108.206914, -27.274116) ccw
  ellipse E395 centre (-108.256061, -25.099818) end of major axis (-108.249636, -24.909926) minor radius 0.079929 (-108.2655, -24.913115) -> (-108.335644, -25.134578) ccw
  line L533 (-108.071665, -24.573622) -> (-108.141216, -23.197921)
  line L534 (-108.230239, -23.045979) -> (-109.143356, -23.444812)
  line L535 (-108.84528, -29.340672) -> (-107.932163, -28.94184)
  line L536 (-107.862018, -28.720377) -> (-107.931569, -27.344676)
  line L537 (-107.935661, -24.578223) -> (-108.005212, -23.202522)
  line L538 (-107.726014, -28.724978) -> (-107.795566, -27.349278)
  line L539 (-108.709276, -29.345274) -> (-107.796159, -28.946441)
  ellipse E396 centre (-108.2208, -23.232682) end of major axis (-108.214375, -23.04279) minor radius 0.079929 (-108.141216, -23.197921) -> (-108.230239, -23.045979) ccw
  ellipse E397 centre (-107.941602, -28.755138) end of major axis (-107.948026, -28.945029) minor radius 0.079929 (-107.932163, -28.94184) -> (-107.862018, -28.720377) ccw
  ellipse E398 centre (-108.084796, -23.237283) end of major axis (-108.078371, -23.047392) minor radius 0.079929 (-108.005212, -23.202522) -> (-108.078371, -23.047392) ccw
  ellipse E399 centre (-107.805598, -28.759739) end of major axis (-107.812023, -28.94963) minor radius 0.079929 (-107.796159, -28.946441) -> (-107.726014, -28.724978) ccw
  line L540 (-108.214375, -23.04279) -> (-108.078371, -23.047392)
  line L541 (-107.645327, -29.430551) -> (-108.587319, -29.39868)
  line L542 (-108.650148, -29.426123) -> (-107.64383, -29.46017)
  ellipse E400 centre (-108.482604, -29.352943) end of major axis (-108.732285, -29.365566) minor radius 0.044682 (-108.709276, -29.345274) -> (-108.587319, -29.39868) ccw
  ellipse E401 centre (-108.78068, -23.457082) end of major axis (-109.180169, -23.477279) minor radius 0.071491 (-109.143356, -23.444812) -> (-109.180169, -23.477279) ccw
  ellipse E402 centre (-108.482604, -29.352943) end of major axis (-108.882093, -29.37314) minor radius 0.071491 (-108.84528, -29.340672) -> (-108.650148, -29.426123) ccw
  line L543 (-109.180169, -23.477279) -> (-109.09174, -25.226384)
  line L544 (-108.970523, -27.624034) -> (-108.882093, -29.37314)
  ellipse E403 centre (-87.38426, -24.498865) end of major axis (-87.360616, -24.687388) minor radius 0.095931 (-87.362972, -24.687626) -> (-87.28852, -24.491583) ccw
  line L545 (-87.360616, -24.687388) -> (-87.387168, -24.690719)
  line L546 (-87.562194, -24.702779) -> (-87.362972, -24.687626)
  line L547 (-87.20605, -27.120563) -> (-87.402003, -27.135468)
  line L548 (-87.519031, -26.95399) -> (-87.619191, -26.06588)
  line L549 (-87.28852, -24.491583) -> (-87.445379, -23.100718)
  line L550 (-87.562407, -22.91924) -> (-87.768742, -22.934934)
  line L551 (-87.988644, -28.963645) -> (-87.047777, -28.89208)
  line L552 (-88.060131, -28.975423) -> (-87.429157, -28.927429)
  ellipse E404 centre (-87.541119, -23.108) end of major axis (-87.564763, -22.919477) minor radius 0.095931 (-87.445379, -23.100718) -> (-87.562407, -22.91924) ccw
  ellipse E405 centre (-87.423291, -26.946708) end of major axis (-87.399647, -27.135231) minor radius 0.095931 (-87.519031, -26.95399) -> (-87.402003, -27.135468) ccw
  ellipse E406 centre (-88.331231, -29.006611) end of major axis (-88.728711, -29.051439) minor radius 0.00852 (-87.988644, -28.963645) -> (-88.059264, -28.969701) ccw
  line L553 (-106.234762, -22.938548) -> (-106.337356, -22.931826)
  line L554 (-106.861544, -28.902377) -> (-106.109341, -28.951659)
  line L555 (-106.009589, -28.76804) -> (-105.994567, -28.634837)
  line L556 (-106.546273, -28.93077) -> (-105.973767, -28.968278)
  line L557 (-106.536792, -24.700212) -> (-106.441319, -24.706467)
  line L558 (-106.376199, -26.116637) -> (-106.470902, -26.956364)
  line L559 (-106.570654, -27.139984) -> (-106.810175, -27.124291)
  ellipse E407 centre (-106.175261, -24.744529) end of major axis (-106.572741, -24.699702) minor radius 0.00852 (-106.536792, -24.700212) -> (-106.563897, -24.698921) ccw
  ellipse E408 centre (-106.448644, -27.168608) end of major axis (-106.846124, -27.123781) minor radius 0.00852 (-106.810175, -27.124291) -> (-106.846124, -27.123781) ccw
  ellipse E409 centre (-106.549366, -26.951223) end of major axis (-106.572483, -27.139812) minor radius 0.078528 (-106.570654, -27.139984) -> (-106.470902, -26.956364) ccw
  ellipse E410 centre (-106.088053, -28.762899) end of major axis (-106.111171, -28.951487) minor radius 0.078528 (-106.109341, -28.951659) -> (-106.009589, -28.76804) ccw
  ellipse E411 centre (-105.952479, -28.779518) end of major axis (-105.975597, -28.968106) minor radius 0.078528 (-105.973767, -28.968278) -> (-105.945508, -28.95855) ccw
  ellipse E412 centre (-105.975825, -22.976143) end of major axis (-106.373305, -22.931316) minor radius 0.00852 (-106.337356, -22.931826) -> (-106.373305, -22.931316) ccw
  line L560 (-106.373305, -22.931316) -> (-106.376412, -22.958864)
  line L561 (-106.846124, -27.123781) -> (-106.847309, -27.134289)
  ellipse E413 centre (-85.030963, -25.055176) end of major axis (-85.093823, -25.234477) minor radius 0.159857 (-85.040403, -25.241878) -> (-84.942903, -25.200882) ccw
  ellipse E414 centre (-85.107471, -25.028354) end of major axis (-85.170331, -25.207654) minor radius 0.159857 (-85.116911, -25.215056) -> (-85.026516, -25.179818) ccw
  ellipse E415 centre (-84.963861, -25.011773) end of major axis (-84.952956, -25.20146) minor radius 0.096916 (-84.9733, -25.198475) -> (-84.952956, -25.20146) ccw
  ellipse E416 centre (-84.835055, -25.004368) end of major axis (-84.82415, -25.194055) minor radius 0.096916 (-84.844494, -25.19107) -> (-84.738144, -25.038343) ccw
  ellipse E417 centre (-84.97515, -27.775423) end of major axis (-84.986055, -27.585736) minor radius 0.096916 (-84.87824, -27.809398) -> (-84.965711, -27.58872) ccw
  line L562 (-84.82415, -25.194055) -> (-84.952956, -25.20146)
  line L563 (-85.209166, -25.220359) -> (-85.116911, -25.215056)
  line L564 (-85.040403, -25.241878) -> (-85.256011, -25.254273)
  line L565 (-85.160727, -25.080204) -> (-84.844494, -25.19107)
  line L566 (-84.9733, -25.198475) -> (-85.23025, -25.108392)
  line L567 (-85.95641, -24.801251) -> (-85.660579, -24.904965)
  line L568 (-85.573108, -25.125642) -> (-85.675448, -27.149887)
  line L569 (-85.781797, -27.302614) -> (-86.077628, -27.198901)
  line L570 (-84.965711, -27.58872) -> (-85.281944, -27.477854)
  line L571 (-85.369415, -27.257177) -> (-85.267076, -25.232932)
  ellipse E418 centre (-86.299893, -24.820997) end of major axis (-85.900403, -24.841193) minor radius 0.071491 (-85.95641, -24.801251) -> (-86.389302, -24.746857) ccw
  ellipse E419 centre (-86.299893, -24.820997) end of major axis (-86.549574, -24.808373) minor radius 0.044682 (-86.085216, -24.808656) -> (-86.298921, -24.776307) ccw
  line L572 (-85.789385, -24.912369) -> (-86.085216, -24.808656)
  ellipse E420 centre (-86.421111, -27.218646) end of major axis (-86.8206, -27.198449) minor radius 0.071491 (-86.077628, -27.198901) -> (-86.512979, -27.144489) ccw
  line L573 (-85.804254, -27.157292) -> (-85.701914, -25.133046)
  line L574 (-87.205616, -26.943361) -> (-87.190173, -26.637889)
  line L575 (-87.128539, -25.418801) -> (-87.106789, -24.988584)
  line L576 (-85.326557, -29.361811) -> (-86.357275, -29.421063)
  line L577 (-86.358858, -29.452374) -> (-85.250049, -29.388634)
  ellipse E421 centre (-85.317118, -29.175109) end of major axis (-85.379978, -29.354409) minor radius 0.159857 (-85.326557, -29.361811) -> (-85.236163, -29.326573) ccw
  ellipse E422 centre (-85.24061, -29.201931) end of major axis (-85.30347, -29.381232) minor radius 0.159857 (-85.250049, -29.388634) -> (-85.15255, -29.347637) ccw
  line L578 (-84.738144, -25.038343) -> (-84.668593, -23.662642)
  line L579 (-84.756064, -23.441965) -> (-85.867981, -23.052146)
  line L580 (-86.166057, -28.948006) -> (-85.054141, -29.337825)
  line L581 (-84.947791, -29.185098) -> (-84.87824, -27.809398)
  line L582 (-86.294863, -28.955411) -> (-85.182947, -29.34523)
  ellipse E423 centre (-84.765504, -23.628667) end of major axis (-84.776408, -23.438981) minor radius 0.096916 (-84.668593, -23.662642) -> (-84.756064, -23.441965) ccw
  ellipse E424 centre (-85.044701, -29.151123) end of major axis (-85.033797, -29.34081) minor radius 0.096916 (-85.054141, -29.337825) -> (-84.947791, -29.185098) ccw
  ellipse E425 centre (-85.173507, -29.158528) end of major axis (-85.162603, -29.348215) minor radius 0.096916 (-85.182947, -29.34523) -> (-85.162603, -29.348215) ccw
  line L583 (-85.033797, -29.34081) -> (-85.162603, -29.348215)
  ellipse E426 centre (-85.670018, -25.091667) end of major axis (-85.680923, -24.90198) minor radius 0.096916 (-85.573108, -25.125642) -> (-85.660579, -24.904965) ccw
  ellipse E427 centre (-85.772358, -27.115912) end of major axis (-85.761453, -27.305599) minor radius 0.096916 (-85.781797, -27.302614) -> (-85.675448, -27.149887) ccw
  ellipse E428 centre (-85.272505, -27.291152) end of major axis (-85.261601, -27.480839) minor radius 0.096916 (-85.369415, -27.257177) -> (-85.281944, -27.477854) ccw
  ellipse E429 centre (-85.170166, -25.266907) end of major axis (-85.18107, -25.07722) minor radius 0.096916 (-85.160727, -25.080204) -> (-85.267076, -25.232932) ccw
  ellipse E430 centre (-85.798824, -25.099071) end of major axis (-85.809729, -24.909384) minor radius 0.096916 (-85.701914, -25.133046) -> (-85.789385, -24.912369) ccw
  ellipse E431 centre (-86.866199, -24.987676) end of major axis (-86.803339, -24.808376) minor radius 0.159857 (-87.025585, -24.966252) -> (-87.027369, -24.976764) ccw